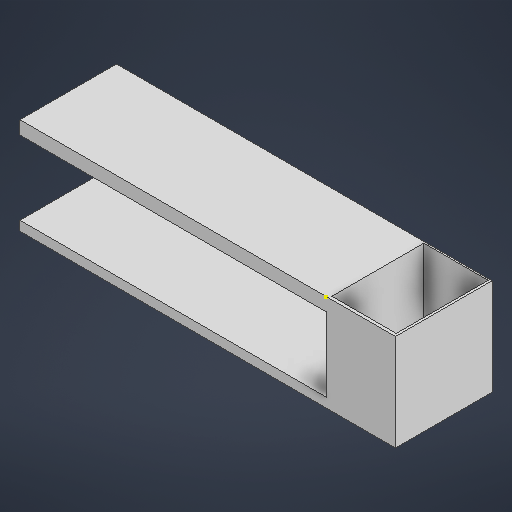
# Autodesk Inventor part: soporte para motor
Saved by Autodesk Inventor 2026.1 (Build 301233020, 233B)
## iProperties
Created: 2025-10-30
Part Number: soporte para motor
Material: Generic
Document SubType Name: Sheet Metal
Designer: Tito Luyo Murata
Density: 1 g/cm^3
Sheet Metal Rule: Default_mm
Appearance: Default
Author: Tito Luyo Murata
Autodesk Inventor part; units mm, degrees
ref_plane "YZ Plane" through (0, 0, 0) normal (1, 0, 0) x (0, 1, 0)
ref_plane "XZ Plane" through (0, 0, 0) normal (0, 1, 0) x (-1, 0, 0)
ref_plane "XY Plane" through (0, 0, 0) normal (0, 0, 1) x (1, 0, 0)
sketch "Sketch7" plane through (0, 0, 0) normal (0, 0, 1) x (1, 0, 0)
  line L0 (0, 0) -> (45, 0)
  line L1 (45, 0) -> (45, -63)
  line L2 (45, -63) -> (0, -63)
  line L3 (0, -63) -> (0, 0)
  dimension "d19" = 45
  dimension "d20" = 63
  constraints: 8 end point, 2 parallel, 1 horizontal, 1 perpendicular
  measures "d19" distance of L1.end L2.end
  measures "d20" distance of L0.end L1.end
extrude "Extrusion3" add sketch "Sketch7" along normal blind 63
sketch "Sketch8" plane through (0, -63, 0) normal (0, -1, 0) x (1, 0, 0)
  line L0 (0, 0) -> (45, 0) projected
  line L1 (1.5, 0) -> (0, 0)
  line L2 (1.5, 1) -> (43.5, 1)
  line L3 (43.5, 1) -> (43.5, 61)
  line L4 (43.5, 61) -> (1.5, 61)
  line L5 (1.5, 61) -> (1.5, 1)
  dimension "d26" = 42
  dimension "d27" = 60
  constraints: 10 end point, 2 parallel, 1 collinear, 1 horizontal, 1 perpendicular, 1 point on line
  measures "d26" distance of L4.end L3.end
  measures "d27" distance of L3.end L2.end
extrude "Extrusion4" cut sketch "Sketch8" against normal blind 63
sketch "Sketch9" plane through (0, 0, 63) normal (0, 0, 1) x (1, 0, 0)
  point P0 (0, 0)
sketch "Sketch10" plane through (0, -63, 0) normal (-1, 0, 0) x (0, 0, 1)
  line L0 (63, 0) -> (63, 63) projected
  line L1 (63, 0) -> (0, 0)
  line L2 (0, 0) -> (0, 6.1882)
  line L3 (0, 6.1882) -> (63, 6.1882)
  line L4 (63, 6.1882) -> (63, 0)
  point P0 (0, 63)
  constraints: 8 end point, 2 parallel, 1 horizontal, 1 perpendicular
extrude "Extrusion5" add sketch "Sketch10" along normal blind 200
sketch "Sketch11" plane through (0, 0, 0) normal (-1, 0, 0) x (0, 0, 1)
  line L0 (63, -63) -> (63, 0) projected
  line L1 (0, 0) -> (0, -56.8118) projected
  line L2 (63, 0) -> (0, 0)
  line L3 (0, 0) -> (0, -8.6425)
  line L4 (0, -8.6425) -> (63, -8.6425)
  line L5 (63, -8.6425) -> (63, 0)
  constraints: 8 end point, 2 parallel, 1 horizontal, 1 perpendicular, 1 point on line
extrude "Extrusion6" add sketch "Sketch11" along normal blind 200
equation "\"BendRadius\" = Thickness"
equation "\"BendReliefWidth\" = Thickness"
equation "\"BendReliefDepth\" = 0.5 * Thickness"
equation "\"CornerReliefSize\" = 4 * Thickness"
equation "\"MinimumRemnant\" = 2 * Thickness"
equation "\"TransitionRadius\" = BendRadius"
equation "\"JacobiRadiusSize\" = BendRadius"
equation "\"GapSize\" = Thickness"
equation "\"Thickness\" = 0.5"
body "Solid2"
